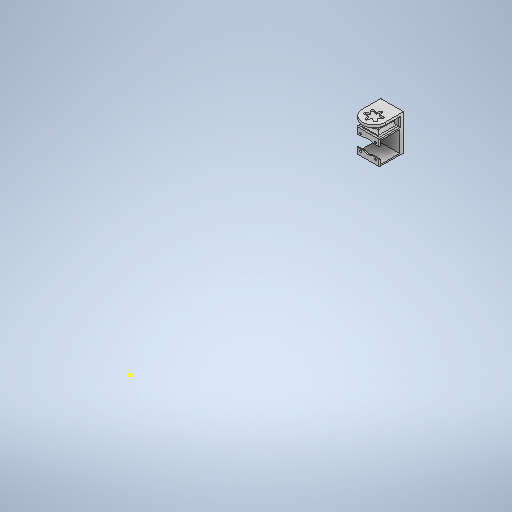
# Autodesk Inventor part: support palonnier test v2
Saved by Autodesk Inventor 2026.2 (Build 302298010, 298A)
## iProperties
Created: 2026-04-23
Part Number: support palonnier test v2
Material: Générique
Document SubType Name: Modeling
Designer: Genon
Density: 1 g/cm^3
Appearance: Par défaut
Author: Genon
Autodesk Inventor part; units mm, degrees
ref_plane "YZ Plane" through (0, 0, 0) normal (1, 0, 0) x (0, 1, 0)
ref_plane "XZ Plane" through (0, 0, 0) normal (0, 1, 0) x (-1, 0, 0)
ref_plane "XY Plane" through (0, 0, 0) normal (0, 0, 1) x (1, 0, 0)
sketch "Esquisse1" plane through (0, 0, 0) normal (1, 0, 0) x (0, 1, 0)
  line L0 (615.5373, -142.1522) -> (811.8285, -142.1522) construction
  line L1 (811.8285, -142.1522) -> (811.8285, -230.5611) construction
  line L2 (811.8285, -230.5611) -> (615.5373, -230.5611) construction
  line L3 (615.5373, -230.5611) -> (615.5373, -142.1522) construction
  circle A0 centre (714.0804, -164.9097) radius 9.3044
  circle A1 centre (714.0804, -164.9097) radius 12.8446
  arc A2 (718.2667, -201.6616) -> (719.1833, -202.8097) centre (719.23, -201.8325) ccw
  arc A3 (719.6606, -209.9141) -> (719.248, -210.7518) centre (719.7361, -210.4718) ccw
  arc A4 (713.6782, -215.3851) -> (712.2032, -215.3703) centre (712.9331, -216.1323) ccw
  line L4 (711.5826, -198.3788) -> (715.3474, -192.8257)
  line L5 (715.3474, -192.8257) -> (719.8038, -195.0511)
  line L6 (719.8038, -195.0511) -> (718.2667, -201.6616)
  line L7 (719.1833, -202.8097) -> (725.8864, -202.9912)
  line L8 (725.8864, -202.9912) -> (726.1597, -208.1294)
  line L9 (726.1597, -208.1294) -> (719.6606, -209.9141)
  line L10 (719.248, -210.7518) -> (722.051, -216.9958)
  line L11 (722.051, -216.9958) -> (717.7376, -219.4332)
  line L12 (717.7376, -219.4332) -> (713.6782, -215.3851)
  line L13 (712.2032, -215.3703) -> (708.5343, -221.0039)
  line L14 (708.5343, -221.0039) -> (704.0426, -218.7609)
  line L15 (704.0426, -218.7609) -> (705.4927, -212.5247)
  line L16 (704.6548, -211.4369) -> (698.081, -211.076)
  line L17 (698.081, -211.076) -> (698.1175, -205.8223)
  line L18 (698.1175, -205.8223) -> (703.9597, -204.218)
  line L19 (704.461, -202.9923) -> (701.4433, -196.9238)
  line L20 (701.4433, -196.9238) -> (705.5988, -194.2119)
  line L21 (705.5988, -194.2119) -> (709.8549, -198.4562)
  arc A5 (719.8038, -195.0511) -> (715.3474, -192.8257) centre (717.4272, -194.2357) ccw
  arc A6 (726.1597, -208.1294) -> (725.8864, -202.9912) centre (725.4624, -205.5902) ccw
  arc A7 (717.7376, -219.4332) -> (722.051, -216.9958) centre (719.7814, -218.0147) ccw
  arc A8 (704.0426, -218.7609) -> (708.5343, -221.0039) centre (706.417, -219.625) ccw
  arc A9 (698.1175, -205.8223) -> (698.081, -211.076) centre (698.2252, -208.45) ccw
  arc A10 (705.5988, -194.2119) -> (701.4433, -196.9238) centre (703.68, -195.8115) ccw
  arc A11 (709.8549, -198.4562) -> (711.5826, -198.3788) centre (710.6833, -197.6255) ccw
  arc A12 (703.9597, -204.218) -> (704.461, -202.9923) centre (703.6717, -203.3848) ccw
  arc A13 (705.4927, -212.5247) -> (704.6548, -211.4369) centre (704.6286, -212.3238) ccw
  point P0 (0, 0)
  constraints: 38 end point, 24 point on circle, 14 centre point, 10 tangent, 4 parallel, 1 coincident, 2 other
extrude "Extrusion1" add sketch "Esquisse1" against normal blind 3 contours A2 L7 L8 L9 A3 L10 L11 L12 A4 L13 L14 L15 A13 L16 L17 L18 A12 L19 L20 L21 A11 L4 L5 L6 | L5 A5 | A6 L8 | L20 A10 | A7 L11 | L17 A9 | A8 L14
sketch "Esquisse2" plane through (0, 0, 0) normal (1, 0, 0) x (0, 0, -1)
  circle A0 centre (207.0147, 711.4157) radius 23.5
  arc A1 (198.4562, 709.8549) -> (198.3788, 711.5826) centre (197.6255, 710.6833) ccw projected
  line L0 (198.3788, 711.5826) -> (192.8257, 715.3474) projected
  arc A2 (195.0511, 719.8038) -> (192.8257, 715.3474) centre (194.2357, 717.4272) ccw projected
  line L1 (195.0511, 719.8038) -> (201.6616, 718.2667) projected
  arc A3 (201.6616, 718.2667) -> (202.8097, 719.1833) centre (201.8325, 719.23) ccw projected
  line L2 (202.8097, 719.1833) -> (202.9912, 725.8864) projected
  arc A4 (208.1294, 726.1597) -> (202.9912, 725.8864) centre (205.5902, 725.4624) ccw projected
  line L3 (208.1294, 726.1597) -> (209.9141, 719.6606) projected
  arc A5 (209.9141, 719.6606) -> (210.7518, 719.248) centre (210.4718, 719.7361) ccw projected
  line L4 (210.7518, 719.248) -> (216.9958, 722.051) projected
  arc A6 (219.4332, 717.7376) -> (216.9958, 722.051) centre (218.0147, 719.7814) ccw projected
  line L5 (219.4332, 717.7376) -> (215.3851, 713.6782) projected
  arc A7 (215.3851, 713.6782) -> (215.3703, 712.2032) centre (216.1323, 712.9331) ccw projected
  line L6 (215.3703, 712.2032) -> (221.0039, 708.5343) projected
  arc A8 (218.7609, 704.0426) -> (221.0039, 708.5343) centre (219.625, 706.417) ccw projected
  line L7 (218.7609, 704.0426) -> (212.5247, 705.4927) projected
  arc A9 (212.5247, 705.4927) -> (211.4369, 704.6548) centre (212.3238, 704.6286) ccw projected
  line L8 (211.4369, 704.6548) -> (211.076, 698.081) projected
  arc A10 (205.8223, 698.1175) -> (211.076, 698.081) centre (208.45, 698.2252) ccw projected
  line L9 (205.8223, 698.1175) -> (204.218, 703.9597) projected
  arc A11 (204.218, 703.9597) -> (202.9923, 704.461) centre (203.3848, 703.6717) ccw projected
  line L10 (202.9923, 704.461) -> (196.9238, 701.4433) projected
  arc A12 (194.2119, 705.5988) -> (196.9238, 701.4433) centre (195.8115, 703.68) ccw projected
  line L11 (194.2119, 705.5988) -> (198.4562, 709.8549) projected
  line L12 (208.4318, 695.5954) -> (205.4503, 728.092)
  line L13 (220.1807, 721.0053) -> (193.7195, 702.3148)
  line L14 (222.0156, 705.5988) -> (191.9877, 718.5497)
  point P0 (0, 0)
  dimension "d12" = 47
  constraints: 6 end point, 6 point on circle, 1 centre point
  measures "d12" diameter of A0
extrude "Extrusion2" add sketch "Esquisse2" against normal blind 6
sketch "Esquisse5" plane through (0, 711.4157, -207.0147) normal (1, 0, 0) x (0, 0, -1)
  point P0 (-207.0147, -711.4157)
ref_plane "Plan de construction1" through (0, 711.4157, -207.0147) normal (1, 0, 0) x (0, 0, -1)
sketch "Esquisse6" plane through (0, 711.4157, -207.0147) normal (1, 0, 0) x (0, 0, -1)
  circle A0 centre (0, 0) radius 23.5 projected
  line L0 (-23.5, 0) -> (-23.5, 40)
  line L1 (-23.5, 0) -> (16.5, 0) construction
  line L2 (-23.5, 40) -> (23.5, 40)
  line L3 (23.5, 40) -> (23.5, 0)
  point P0 (-207.0147, -711.4157)
  dimension "d14" = 40
  dimension "d15" = 90
  constraints: 8 end point, 2 perpendicular, 2 point on circle, 2 tangent, 1 horizontal, 1 vertical
  measures "d14" distance of L0.start L0.end
  measures "d15" angle of L1 L0
extrude "Extrusion3" add sketch "Esquisse6" against normal blind 6 contours A0 L0 L2 L3
sketch "Esquisse7" plane through (0, 0, 0) normal (1, 0, 0) x (0, 0, -1)
  arc A0 (183.5147, 711.4157) -> (230.5147, 711.4157) centre (207.0147, 711.4157) ccw projected
  line L0 (230.5147, 711.4157) -> (230.5147, 751.4157) projected
  line L1 (230.5147, 751.4157) -> (183.5147, 751.4157) projected
  line L2 (183.5147, 751.4157) -> (183.5147, 711.4157) projected
  line L3 (183.5147, 711.4157) -> (183.5147, 751.4157) projected
  line L4 (183.5147, 751.4157) -> (183.5147, 741.4157)
  line L5 (183.5147, 741.4157) -> (230.5147, 741.4157)
  point P0 (0, 0)
  dimension "d18" = 10
  constraints: 4 end point, 2 point on line, 1 perpendicular
  measures "d18" distance of L1.end L4.end
extrude "Extrusion4" add sketch "Esquisse7" along normal blind 70 contours L2 L1 L0 L5
sketch "Esquisse8" plane through (0, 741.4157, -230.5147) normal (0, -1, 0) x (1, 0, 0)
  line L0 (70, 47) -> (70, 0) projected
  line L1 (70, 0) -> (65, 0)
  line L2 (0, 0) -> (70, 0) projected
  line L3 (65, 0) -> (65, 47)
  line L4 (65, 47) -> (70, 47)
  point P0 (0, 230.5147)
  dimension "d21" = 5
  constraints: 6 end point, 2 perpendicular, 1 point on line
  measures "d21" distance of L0.end L1.end
extrude "Extrusion5" add sketch "Esquisse8" along normal blind 40
ref_plane "Plan de construction2" through (22, 0, 0) normal (1, 0, 0) x (0, 0, -1)
ref_plane "Plan de construction3" through (0, 741.4157, -230.5147) normal (0, -1, 0) x (1, 0, 0)
sketch "Esquisse9" plane through (0, 741.4157, -230.5147) normal (0, -1, 0) x (1, 0, 0)
  line L0 (70, 0) -> (70, 47) projected
  line L1 (70, 0) -> (22, 0)
  line L2 (70, 0) -> (-6, 0) projected
  line L3 (22, 0) -> (22, 47)
  line L4 (22, 47) -> (17, 47)
  line L5 (17, 47) -> (17, 0)
  line L6 (22, 0) -> (17, 0)
  point P0 (0, 230.5147)
  dimension "d26" = 48
  dimension "d27" = 47
  dimension "d28" = 5
  constraints: 10 end point, 3 perpendicular, 2 point on line, 1 collinear
  measures "d26" distance of L0.start L1.end
  measures "d27" distance of L1.end L3.end
  measures "d28" distance of L3.end L4.end
extrude "Extrusion6" add sketch "Esquisse9" along normal blind 40
sketch "Esquisse10" plane through (0, 701.4157, -230.5147) normal (0, -1, 0) x (1, 0, 0)
  line L0 (17, 47) -> (17, 0) projected
  line L1 (70, 0) -> (70, 47) projected
  line L2 (-6, 47) -> (70, 47) projected
  line L3 (17, 0) -> (32, 0)
  line L4 (32, 0) -> (32, 47)
  line L5 (32, 47) -> (17, 47)
  line L6 (17, 47) -> (17, 0)
  line L7 (70, 0) -> (55, 0)
  line L8 (55, 0) -> (55, 47)
  line L9 (55, 47) -> (70, 47)
  line L10 (70, 47) -> (70, 0)
  point P0 (0, 230.5147)
  dimension "d31" = 15
  dimension "d32" = 15
  constraints: 16 end point, 4 parallel, 2 horizontal, 2 perpendicular, 1 midpoint, 1 point on line
  measures "d31" distance of L5.end L4.end
  measures "d32" distance of L8.end L9.end
extrude "Extrusion7" add sketch "Esquisse10" along normal blind 1.75
sketch "Esquisse11" plane through (0, 699.6657, -230.5147) normal (0, -1, 0) x (1, 0, 0)
  line L0 (22, 47) -> (22, 0) projected
  line L1 (65, 0) -> (65, 47) projected
  line L2 (22, 23.5) -> (65, 23.5)
  circle A0 centre (43.5, 23.5) radius 14
  point P0 (0, 230.5147)
  dimension "d35" = 28
  constraints: 3 midpoint, 2 end point, 1 centre point
  measures "d35" diameter of A0
extrude "Extrusion8" cut sketch "Esquisse11" against normal blind 1.75
sketch "Esquisse12" plane through (0, 699.6657, -230.5147) normal (0, -1, 0) x (1, 0, 0)
  line L0 (65, 47) -> (65, 0) projected
  line L1 (65, 0) -> (59.3, 0)
  line L2 (55, 0) -> (70, 0) projected
  line L3 (59.3, 0) -> (59.3, 23.5)
  line L4 (59.3, 23.5) -> (59.3, 39)
  line L5 (59.3, 23.5) -> (59.3, 8)
  line L6 (59.3, 8) -> (28.3, 8)
  line L7 (28.3, 8) -> (28.3, 39)
  point P0 (0, 230.5147)
  dimension "d38" = 5.7
  dimension "d39" = 23.5
  dimension "d40" = 15.5
  dimension "d41" = 15.5
  dimension "d42" = 31
  constraints: 12 end point, 4 coincident, 3 point on line, 2 perpendicular, 1 parallel
  measures "d38" distance of L0.end L1.end
  measures "d39" distance of L1.end L3.end
  measures "d40" distance of L3.end L4.end
  measures "d41" distance of L3.end L5.end
  measures "d42" distance of L5.end L6.end
hole "Perçage1" at (28.3, 699.6657, -222.5147) at (28.3, 699.6657, -191.5147) at (59.3, 699.6657, -191.5147) at (59.3, 699.6657, -222.5147) direction (0, 1, 0) diameter 4.5 depth 8.8 tip angle 118
sketch "Esquisse13" plane through (0, 0, 0) normal (1, 0, 0) x (0, 0, -1)
  line L0 (230.5147, 741.4157) -> (183.5147, 741.4157) projected
  line L1 (183.5147, 741.4157) -> (183.5147, 711.4157) projected
  arc A0 (183.5147, 711.4157) -> (230.5147, 711.4157) centre (207.0147, 711.4157) ccw projected
  line L2 (230.5147, 711.4157) -> (230.5147, 741.4157) projected
  point P0 (0, 0)
extrude "Extrusion9" add sketch "Esquisse13" along normal blind 1
sketch "Esquisse14" plane through (17, 699.6657, -230.5147) normal (-1, 0, 0) x (0, 0, 1)
  line L0 (0, 41.75) -> (47, 41.75) projected
  line L1 (47, 41.75) -> (23.5, 41.75)
  line L2 (23.5, 41.75) -> (23.5, 20.875)
  line L3 (35.5, 32.875) -> (11.5, 32.875)
  line L4 (11.5, 32.875) -> (11.5, 8.875)
  line L5 (11.5, 8.875) -> (35.5, 8.875)
  line L6 (35.5, 8.875) -> (35.5, 32.875)
  line L7 (35.5, 32.875) -> (11.5, 8.875) construction
  line L8 (11.5, 32.875) -> (35.5, 8.875) construction
  line L9 (47, 41.75) -> (0, 41.75) projected
  line L10 (11.5, 32.875) -> (35.5, 32.875)
  line L11 (35.5, 32.875) -> (35.5, 41.75)
  line L12 (35.5, 41.75) -> (11.5, 41.75)
  line L13 (11.5, 41.75) -> (11.5, 32.875)
  point P0 (230.5147, -699.6657)
  point P1 (11.5, 41.75)
  point P2 (35.5, 32.875)
  point P3 (35.5, 41.75)
  dimension "d53" = 20.875
  dimension "d54" = 24
  dimension "d55" = 24
  constraints: 24 end point, 4 parallel, 3 midpoint, 3 perpendicular, 2 horizontal, 1 point on line
  measures "d53" distance of L1.end L2.end
  measures "d54" distance of L5.end L4.end
  measures "d55" distance of L4.end L3.end
extrude "Extrusion10" add sketch "Esquisse14" along normal up to surface (16 mm away)
fillet "Congé2" radius 5 2 edges at (17, 724.9782, -195.0147) (17, 708.5407, -207.0147)
fillet "Congé3" radius 2 8 edges at (24.5, 699.6657, -230.5147) (17, 699.6657, -207.0147) (1, 726.4157, -230.5147) (1, 687.9157, -207.0147) (1, 726.4157, -183.5147) (17, 720.5407, -183.5147) (17, 720.5407, -230.5147) (24.5, 699.6657, -183.5147)
fillet "Congé4" radius 2 5 edges at (62.5, 699.6657, -183.5147) (70, 725.5407, -183.5147) (70, 699.6657, -207.0147) (62.5, 699.6657, -230.5147) (70, 725.5407, -230.5147)
fillet "Congé5" radius 2 6 edges at (-6, 751.4157, -207.0147) (69.4142, 751.4157, -184.1004) (31, 751.4157, -183.5147) (69.4142, 751.4157, -229.9289) (31, 751.4157, -230.5147) (70, 751.4157, -207.0147)
fillet "Congé6" radius 5 5 edges at (1, 708.5407, -207.0147) (1, 724.9782, -195.0147) (1, 724.9782, -219.0147) (17, 706.0407, -219.0147) (17, 724.9782, -219.0147)
ref_plane "Plan de construction4" through (-4, 711.4157, -228.5147) normal (0, 1, 0) x (1, 0, 0)
fillet "Congé7" radius 2 6 edges at (0, 741.4157, -183.5147) (9, 741.4157, -183.5147) (18, 741.4157, -183.5147) (18, 741.4157, -230.5147) (9, 741.4157, -230.5147) (0, 741.4157, -230.5147)
